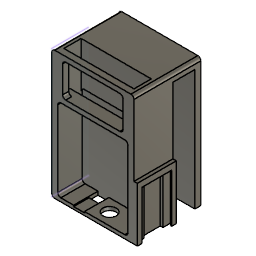
electronics_holder (Autodesk Fusion 360 design; units mm, degrees)
Autodesk Fusion 360 part; units mm, degrees
sketch "Sketch1" plane through (0, 0, 0) normal (0, 0, 1) x (1, 0, 0)
  line L0 (28.775, -7.5) -> (-28.775, -7.5)
  line L1 (-28.775, -7.5) -> (-28.775, 7.5)
  line L2 (-28.775, 7.5) -> (28.775, 7.5)
  line L3 (28.775, 7.5) -> (28.775, -7.5)
  line L4 (28.775, -7.5) -> (-28.775, 7.5) construction
  line L5 (-28.775, -7.5) -> (28.775, 7.5) construction
  line L6 (33.775, -17.5) -> (-33.775, -17.5)
  line L7 (-33.775, -17.5) -> (-33.775, 17.5)
  line L8 (-33.775, 17.5) -> (33.775, 17.5)
  line L9 (33.775, 17.5) -> (33.775, -17.5)
  line L10 (33.775, -17.5) -> (-33.775, 17.5) construction
  line L11 (-33.775, -17.5) -> (33.775, 17.5) construction
  line L12 (-28.775, -7.5) -> (-28.775, -17.5)
  line L13 (28.775, -7.5) -> (28.775, -17.5)
  line L14 (33.775, -7.5) -> (-33.775, -7.5)
  dimension "d1" = 57.55
  dimension "d2" = 15
  dimension "d3" = 10
  dimension "d4" = 5
  constraint horizontal L0
  constraint perpendicular L0 L1
  constraint parallel L0 L2
  constraint parallel L1 L3
  constraint coincident L4 origin
  constraint coincident L5 origin
  constraint horizontal L6
  constraint perpendicular L6 L7
  constraint parallel L6 L8
  constraint parallel L7 L9
  constraint coincident L10 origin
  constraint coincident L11 origin
  constraint coincident L6 L12.end
  constraint perpendicular L6 L12
  constraint coincident L6 L13.end
  constraint perpendicular L6 L13
  constraint coincident L9 L14.start
  constraint coincident L7 L14.end
  constraint perpendicular L7 L14
  measures "d1" distance of L1.end L2.end
  measures "d2" distance of L0.start L2.end
  measures "d3" distance of L2 L8
  measures "d4" distance of L3 L9
extrude "Extrude1" add sketch "Sketch1" against normal blind 5 contours L0 L1 L2 L3 L14 | L1 L2 L3 L7 L8 L9 L14 makes body 1
extrude "Extrude2" add sketch "Sketch1" along normal blind 65.5 contours L1 L2 L3 L7 L8 L9 L14 bodies 1
sketch "Sketch2" plane through (0, 0, 0) normal (0, 0, 1) x (-1, 0, 0)
  line L0 (-28.775, 7.5) -> (-28.775, -7.5)
  line L1 (-28.775, -7.5) -> (28.775, -7.5)
  line L2 (28.775, -7.5) -> (28.775, 7.5)
  line L3 (28.775, 2.5) -> (-28.775, 2.5) construction
  circle A0 centre (-3.775, 2.5) radius 5.25
  line L4 (28.775, 7.5) -> (-28.775, 7.5)
  dimension "d9" = 10.5
  dimension "d10" = 25
  dimension "d11" = 10
  constraint coincident L2 L3.start
  constraint coincident L0 L3.end
  constraint perpendicular L0 L3
  constraint coincident L3 A0.centre
  measures "d9" diameter of A0
  measures "d10" distance of L0 A0.centre
  measures "d11" distance of L1 A0.centre
extrude "Extrude3" cut sketch "Sketch2" against normal blind 10 contours A0 L4 | A0 L4 bodies 1
sketch "Sketch3" plane through (0, 0, 0) normal (0, 0, 1) x (-1, 0, 0)
  line L0 (-28.775, 7.5) -> (-28.775, -7.5)
  line L1 (-28.775, -7.5) -> (28.775, -7.5)
  line L2 (28.775, -7.5) -> (28.775, 7.5)
  line L3 (6.775, -7.5) -> (6.775, -0.1264)
  line L4 (6.775, -0.1264) -> (15.775, -0.1264)
  line L5 (15.775, -0.1264) -> (15.775, -7.5)
  line L6 (28.775, 7.5) -> (-2.1742, 7.5)
  line L7 (-5.3758, 7.5) -> (-28.775, 7.5)
  arc A0 (-5.3758, 7.5) -> (-2.1742, 7.5) centre (-3.775, 2.5) ccw
  dimension "d14" = 13
  dimension "d15" = 9
  constraint coincident L1 L3.start
  constraint perpendicular L1 L3
  constraint perpendicular L3 L4
  constraint coincident L1 L5.end
  constraint perpendicular L1 L5
  measures "d14" distance of L2 L5
  measures "d15" distance of L3.end L4.end
extrude "Extrude4" cut sketch "Sketch3" against normal blind 6 contours L1 L3 L4 L5 bodies 1
sketch "Sketch4" plane through (28.775, 0, 0) normal (-1, 0, 0) x (0, -1, 0)
  line L0 (-7.5, 0) -> (7.5, 0)
  line L1 (7.5, 65.5) -> (-7.5, 65.5)
  line L2 (-7.5, 65.5) -> (-7.5, 0)
  line L3 (-17.5, 65.5) -> (-12.5, 100.5)
  line L4 (-12.5, 100.5) -> (-1.5, 100.5)
  line L5 (-1.5, 100.5) -> (-1.5, 65.5)
  line L6 (-17.5, 65.5) -> (-1.5, 65.5)
  line L7 (7.5, 0) -> (7.5, 65.5)
  point P0 (-17.5, 65.5)
  dimension "d19" = 6
  dimension "d20" = 35
  constraint perpendicular L2 L4
  constraint coincident P0 L3.start
  constraint coincident L1 L5.end
  constraint perpendicular L1 L5
  measures "d19" distance of L1.end L5.end
  measures "d20" distance of L4.end L5.end
extrude "Extrude5" add sketch "Sketch4" along normal blind 57.55 separate body contours L1 L3 L4 L5 L6 makes body 2
extrude "Extrude6" add 1 faces at (9.5917, 14.1667, 65.5) along direction (0, 0, 1) blind 35 on bodies 1 bodies 1 2
sketch "Sketch6" plane through (0, -7.5, 0) normal (0, -1, 0) x (1, 0, 0)
  line L0 (28.775, 0) -> (-28.775, 0)
  line L1 (-28.775, 0) -> (-28.775, 100.5)
  line L2 (-28.775, 100.5) -> (-33.775, 100.5)
  line L3 (-33.775, 100.5) -> (-33.775, -5)
  line L4 (-33.775, -5) -> (33.775, -5)
  line L5 (33.775, -5) -> (33.775, 100.5)
  line L6 (33.775, 100.5) -> (28.775, 100.5)
  line L7 (28.775, 100.5) -> (28.775, 0)
  line L8 (28.775, 65.5) -> (28.775, 100.5)
  line L9 (28.775, 100.5) -> (-28.775, 100.5)
  line L10 (-28.775, 100.5) -> (-28.775, 65.5)
  line L11 (-28.775, 65.5) -> (28.775, 65.5)
  line L12 (-28.775, 100.5) -> (28.775, 65.5) construction
  line L13 (24.775, 69.5) -> (-24.775, 69.5)
  line L14 (-24.775, 69.5) -> (-24.775, 96.5)
  line L15 (-24.775, 96.5) -> (24.775, 96.5)
  line L16 (24.775, 96.5) -> (24.775, 69.5)
  line L17 (24.775, 69.5) -> (-24.775, 96.5) construction
  line L18 (-24.775, 69.5) -> (24.775, 96.5) construction
  line L19 (5.3758, -5) -> (33.775, -5)
  line L20 (33.775, -5) -> (33.775, 100.5)
  line L21 (33.775, 100.5) -> (28.775, 100.5)
  line L22 (28.775, 100.5) -> (28.775, 0)
  line L23 (28.775, 0) -> (5.3758, 0)
  line L24 (5.3758, 0) -> (5.3758, -5)
  point P0 (0, 83)
  dimension "d27" = 4
  dimension "d28" = 4
  constraint coincident L1.end L2.start
  constraint coincident L8.start L11.end
  constraint horizontal L13
  constraint perpendicular L13 L14
  constraint parallel L13 L15
  constraint parallel L14 L16
  constraint coincident L17 P0
  constraint coincident L18 P0
  constraint midpoint L12 P0
  measures "d27" distance of L9 L15
  measures "d28" distance of L7 L16
extrude "Extrude7" add sketch "Sketch6" along normal blind 5 contours L0 L4 L5 L6 L7 L8 L19 L20 L21 L22 L23 L24 | L0 L1 L2 L3 L4 L10 L24 | L1 L7 L8 L9 L10 L11 L22 bodies 1
sketch "Sketch15" plane through (0, -7.5, 0) normal (0, 1, 0) x (-1, 0, 0)
  line L0 (-28.775, 100.5) -> (-28.775, 65.5)
  line L1 (-28.775, 65.5) -> (28.775, 65.5)
  line L2 (28.775, 65.5) -> (28.775, 100.5)
  line L3 (28.775, 100.5) -> (-28.775, 100.5)
  line L4 (-24.775, 96.5) -> (24.775, 96.5)
  line L5 (24.775, 96.5) -> (24.775, 69.5)
  line L6 (24.775, 69.5) -> (-24.775, 69.5)
  line L7 (-24.775, 69.5) -> (-24.775, 96.5)
  line L8 (-24.775, 69.5) -> (-28.775, 69.5)
  line L9 (-28.775, 69.5) -> (28.775, 69.5)
  constraint coincident L6.end L7.start
  constraint coincident L0 L8.end
  constraint perpendicular L0 L8
  constraint coincident L2 L9.end
  constraint perpendicular L2 L9
extrude "Extrude17" add sketch "Sketch15" along normal blind 5 contours L0 L1 L2 L6 L8 L9 bodies 1
fillet "Fillet1" radius 2.5 10 edges at (-24.775, -10, 96.5) (-24.775, -10, 69.5) (24.775, -10, 69.5) (24.775, -10, 96.5) (-28.775, 4.5, 65.5) (-28.775, -10, 65.5) (-28.775, -2.5, 0) (28.775, -2.5, 0) (28.775, -10, 65.5) (28.775, 4.5, 65.5) on bodies 1
sketch "Sketch7" plane through (33.775, 0, 0) normal (1, 0, 0) x (0, 1, 0)
  line L0 (17.5, -5) -> (17.5, 100.5)
  line L1 (-12.5, 100.5) -> (-12.5, -5)
  line L2 (2.5, -4.4234) -> (2.5, 39.7315) construction
  line L3 (-11.625, 39.7315) -> (16.625, 39.7315)
  line L4 (-11.625, 39.7315) -> (-11.625, -5)
  line L5 (16.625, 39.7315) -> (16.618, -5)
  line L6 (-11.625, 39.7315) -> (-12.5, 39.7315)
  line L7 (16.625, 39.7315) -> (17.5, 39.7315)
  line L8 (-12.5, 37) -> (17.5, 37)
  line L9 (-12.5, -5) -> (17.5, -5)
  line L10 (17.5, 100.5) -> (-12.5, 100.5)
  point P0 (2.5, 37)
  dimension "d35" = 28.25
  dimension "d44" = 42
  constraint midpoint L2.end L3
  constraint perpendicular L2 L3
  constraint perpendicular L3 L4
  constraint coincident L1 L6.end
  constraint perpendicular L1 L6
  constraint coincident L0 L7.end
  constraint perpendicular L0 L7
  constraint midpoint L8 P0
  constraint coincident L2 P0
  constraint coincident L0 L8.end
  constraint perpendicular L0 L8
  constraint vertical L2
  constraint coincident L4.end L9
  constraint coincident L5.end L9
  measures "d35" distance of L3.start L3.end
  measures "d44" distance of L8 L9
extrude "Extrude9" add sketch "Sketch7" along normal blind 1.8 contours L0 L5 L8 L9 | L0 L5 L7 L8 | L3 L4 L5 L8 | L1 L4 L8 L9 | L1 L4 L6 L8 bodies 1
sketch "Sketch8" plane through (35.575, 0, 0) normal (1, 0, 0) x (0, 1, 0)
  line L0 (17.5, 39.7315) -> (-12.5, 39.7315)
  line L1 (-12.5, 39.7315) -> (-12.5, -5)
  line L2 (-11.625, -5) -> (-11.625, 37)
  line L3 (-11.625, 37) -> (16.6246, 37)
  line L4 (16.6246, 37) -> (16.618, -5)
  line L5 (17.5, -5) -> (17.5, 39.7315)
  line L6 (-9.6187, 35.0038) -> (14.6243, 35)
  line L7 (-12.5, -5) -> (-11.625, -5)
  line L8 (16.618, -5) -> (17.5, -5)
  line L9 (14.6243, 35) -> (14.618, -5)
  line L10 (-9.6187, 35.0038) -> (-9.625, -5.0074)
  line L11 (17.5, -5) -> (17.5, 39.7315)
  line L12 (17.5, 39.7315) -> (-12.5, 39.7315)
  line L13 (-12.5, 39.7315) -> (-12.5, -5)
  line L14 (-12.5, -5) -> (-11.625, -5)
  line L15 (-11.625, -5) -> (-11.625, 37)
  line L16 (-11.625, 37) -> (16.6246, 37)
  line L17 (16.6246, 37) -> (16.618, -5)
  line L18 (16.618, -5) -> (17.5, -5)
  line L19 (16.618, -5) -> (-11.625, -5)
  dimension "d45" = 2
  dimension "d46" = 2
  dimension "d47" = 2
  constraint perpendicular L4 L6
  constraint perpendicular L6 L9
  constraint perpendicular L6 L10
  constraint coincident L9.end L19
  measures "d45" horizontal distance of L2.start L10.end
  measures "d46" distance of L9.end L4.end
  measures "d47" vertical distance of L6.end L3.end
sketch "Sketch9" plane through (-33.775, 0, 0) normal (-1, 0, 0) x (0, -1, 0)
  line L0 (12.5, -5) -> (12.5, 100.5)
  line L1 (-17.5, 100.5) -> (-17.5, -5)
  line L2 (-17.5, -5) -> (12.5, -5)
  line L3 (12.5, 100.5) -> (-17.5, 100.5)
sketch "Sketch10" plane through (-33.775, 0, 0) normal (-1, 0, 0) x (0, -1, 0)
  line L0 (-17.5, 100.5) -> (-17.5, -5)
  line L1 (-17.5, -5) -> (-37.5, -5)
  line L2 (-37.5, -5) -> (-37.5, 1.25)
  line L3 (-37.5, 1.25) -> (-19.5, 1.25)
  line L4 (-19.5, 1.25) -> (-19.5, 94.25)
  line L5 (-19.5, 94.25) -> (-37.5, 94.25)
  line L6 (-37.5, 94.25) -> (-37.5, 100.5)
  line L7 (-37.5, 100.5) -> (-17.5, 100.5)
  dimension "d48" = 2
  dimension "d49" = 93
  dimension "d50" = 18
  constraint coincident L0.end L1.start
  constraint perpendicular L0 L1
  constraint perpendicular L1 L2
  constraint perpendicular L2 L3
  constraint perpendicular L3 L4
  constraint perpendicular L4 L5
  constraint perpendicular L5 L6
  constraint coincident L0.start L7.end
  constraint perpendicular L0 L7
  constraint equal L2 L6
  constraint equal L3 L5
  measures "d48" distance of L0 L4
  measures "d49" distance of L3.end L4.end
  measures "d50" distance of L2.end L3.end
extrude "Extrude11" add sketch "Sketch10" against normal blind 67.55 bodies 1
sketch "Sketch11" plane through (-33.775, 0, 0) normal (-1, 0, 0) x (0, -1, 0)
  line L0 (-37.5, -5) -> (12.5, -5)
  line L1 (12.5, -5) -> (12.5, 100.5)
  line L2 (12.5, 100.5) -> (-37.5, 100.5)
  line L3 (-37.5, 100.5) -> (-37.5, 94.25)
  line L4 (-37.5, 94.25) -> (-19.5, 94.25)
  line L5 (-19.5, 94.25) -> (-19.5, 1.25)
  line L6 (-19.5, 1.25) -> (-37.5, 1.25)
  line L7 (-37.5, 1.25) -> (-37.5, -5)
  line L8 (-37.5, 1.25) -> (-37.5, 94.25)
  constraint coincident L6.end L7.start
  constraint coincident L3.end L4.start
extrude "Extrude12" add sketch "Sketch11" against normal blind 5 contours L4 L5 L6 L8 bodies 1
sketch "Sketch12" plane through (33.775, 0, 0) normal (1, 0, 0) x (0, 1, 0)
  line L0 (-12.5, 39.7315) -> (17.5, 39.7315)
  line L1 (17.5, 39.7315) -> (17.5, -5)
  line L2 (17.5, -5) -> (37.5, -5)
  line L3 (37.5, -5) -> (37.5, 1.25)
  line L4 (37.5, 1.25) -> (19.5, 1.25)
  line L5 (19.5, 1.25) -> (19.5, 94.25)
  line L6 (19.5, 94.25) -> (37.5, 94.25)
  line L7 (37.5, 94.25) -> (37.5, 100.5)
  line L8 (37.5, 100.5) -> (-12.5, 100.5)
  line L9 (-12.5, 100.5) -> (-12.5, 39.7315)
  line L10 (19.5, 1.25) -> (17.5, 1.25)
  constraint coincident L4.end L5.start
  constraint coincident L1 L10.end
  constraint perpendicular L1 L10
extrude "Extrude13" cut sketch "Sketch12" against normal blind 19 contours L1 L2 L3 L4 L10 bodies 1
extrude "Extrude14" add 1 faces at (27.4417, 18.8333, 1.25) along direction (0, 0, -1) blind 6.25 on bodies 1 bodies 1
sketch "Sketch13" plane through (0, 37.5, 0) normal (0, 1, 0) x (-1, 0, 0)
  line L0 (-14.775, 1.25) -> (-14.775, -5)
  line L1 (-14.775, -5) -> (33.775, -5)
  line L2 (33.775, -5) -> (33.775, 100.5)
  line L3 (33.775, 100.5) -> (-33.775, 100.5)
  line L4 (-33.775, 100.5) -> (-33.775, 94.25)
  line L5 (-33.775, 94.25) -> (28.775, 94.25)
  line L6 (28.775, 94.25) -> (28.775, 1.25)
  line L7 (28.775, 1.25) -> (-14.775, 1.25)
  line L8 (-33.775, 94.25) -> (-33.775, -5)
  line L9 (-33.775, -5) -> (-14.775, -5)
  constraint coincident L4.end L5.start
  constraint perpendicular L5 L8
  constraint coincident L0.end L1.start
  constraint perpendicular L0 L9
extrude "Extrude15" add sketch "Sketch13" along normal blind 5 bodies 1
sketch "Sketch14" plane through (0, 0, -5) normal (0, 0, -1) x (1, 0, 0)
  line L0 (33.775, -17.5) -> (35.575, -17.5)
  line L1 (35.575, -16.618) -> (33.775, -16.618)
  line L2 (33.775, -16.618) -> (33.775, 11.625)
  line L3 (33.775, 11.625) -> (35.575, 11.625)
  line L4 (35.575, 12.5) -> (-33.775, 12.5)
  line L5 (-33.775, 12.5) -> (-33.775, -42.5)
  line L6 (-33.775, -42.5) -> (33.775, -42.5)
  line L7 (33.775, -37.5) -> (14.775, -37.5)
  line L8 (14.775, -37.5) -> (14.775, -19.5)
  line L9 (14.775, -19.5) -> (33.775, -19.5)
  arc A0 (2.1742, 7.5) -> (5.3758, 7.5) centre (3.775, 2.5) ccw
  line L10 (2.1742, 7.5) -> (5.3758, 7.5)
  line L11 (-15.775, -7.5) -> (-15.775, -0.1264)
  line L12 (-15.775, -0.1264) -> (-6.775, -0.1264)
  line L13 (-6.775, -0.1264) -> (-6.775, -7.5)
  line L14 (-6.775, -7.5) -> (-15.775, -7.5)
  circle A1 centre (3.775, 2.5) radius 5.5
  line L15 (35.575, -17.5) -> (35.575, -16.618)
  line L16 (35.575, 11.625) -> (35.575, 12.5)
  line L17 (33.775, -42.5) -> (33.775, -37.5)
  line L18 (33.775, -19.5) -> (33.775, -17.5)
  dimension "d61" = 11
  constraint concentric A0 A1
  measures "d61" diameter of A1
extrude "Extrude16" cut sketch "Sketch14" against normal blind 5 contours A1 bodies 1
extrude "Extrude18" cut 1 faces at (8.7583, 1.5, 88.8333) along direction (0, 1, 0) blind 5.2 on bodies 1 bodies 1
delete_face "DeleteFace1" 1 faces at (26.8644, -5.8333, 0.0705) on bodies 1
delete_face "DeleteFace2" 1 faces at (-28.7637, -5.8333, 2.2624) on bodies 1
extrude "Extrude19" cut 1 faces at (22.275, -2.5, 0) along direction (0, 0, -1) blind 2 on bodies 1 bodies 1
extrude "Extrude20" add 1 faces at (34.975, 17.5, 24.821) along direction (0, 1, 0) blind 2 and the other way blind 30 on bodies 1 bodies 1
sketch "Sketch16" plane through (35.575, 0, 0) normal (1, 0, 0) x (0, 1, 0)
  line L0 (19.5, 39.7315) -> (-12.5, 39.7315)
  line L1 (-12.5, 39.7315) -> (-12.5, -5)
  line L2 (-12.5, -5) -> (19.5, -5)
  line L3 (19.5, -5) -> (19.5, 39.7315)
  line L4 (3.5, -5) -> (3.5, 37) construction
  line L5 (-10.65, 37) -> (17.65, 37)
  line L6 (-10.65, 37) -> (-10.65, -5)
  line L7 (17.65, 37) -> (17.65, -5)
  dimension "d76" = 42
  dimension "d77" = 28.3
  constraint midpoint L2 L4.start
  constraint perpendicular L2 L4
  constraint midpoint L4.end L5
  constraint perpendicular L3 L5
  constraint coincident L2 L6.end
  constraint perpendicular L2 L6
  constraint coincident L2 L7.end
  constraint perpendicular L2 L7
  measures "d76" distance of L4.start L4.end
  measures "d77" distance of L5.start L5.end
extrude "Extrude21" cut sketch "Sketch16" against normal blind 1.75 contours L2 L5 L6 L7 bodies 1
sketch "Sketch17" plane through (33.825, 0, 0) normal (1, 0, 0) x (0, 1, 0)
  line L0 (-10.65, 37) -> (-10.65, -5)
  line L1 (-10.65, -5) -> (17.65, -5)
  line L2 (17.65, -5) -> (17.65, 37)
  line L3 (17.65, 37) -> (-10.65, 37)
  line L4 (3.5, -5) -> (3.5, 37)
  line L5 (-4.25, 37) -> (11.25, 37)
  line L6 (-4.25, 37) -> (-4.25, -5)
  line L7 (11.25, 37) -> (11.25, -5)
  dimension "d80" = 15.5
  constraint midpoint L1 L4.start
  constraint perpendicular L1 L4
  constraint midpoint L4.end L5
  constraint perpendicular L4 L5
  constraint coincident L1 L6.end
  constraint perpendicular L1 L6
  constraint coincident L1 L7.end
  constraint perpendicular L1 L7
  constraint collinear L3 L5
  measures "d80" distance of L5.start L5.end
extrude "Extrude22" cut sketch "Sketch17" against normal blind 2 contours L1 L3 L4 L5 L6 | L1 L3 L4 L5 L7 bodies 1
sketch "Sketch18" plane through (35.575, 0, 0) normal (1, 0, 0) x (0, 1, 0)
  line L0 (-10.65, -5) -> (-10.65, 37)
  line L1 (-10.65, 37) -> (17.65, 37)
  line L2 (17.65, 37) -> (17.65, -5)
  line L3 (17.65, -5) -> (19.5, -5)
  line L4 (19.5, -5) -> (19.5, 39.7315)
  line L5 (19.5, 39.7315) -> (-12.5, 39.7315)
  line L6 (-12.5, 39.7315) -> (-12.5, -5)
  line L7 (-12.5, -5) -> (-10.65, -5)
  line L8 (-10.65, -5) -> (-8.65, -5)
  line L9 (-8.65, -5) -> (-8.65, 35)
  line L10 (-8.65, 35) -> (15.65, 35)
  line L11 (15.65, 35) -> (15.65, -5)
  line L12 (15.65, -5) -> (17.65, -5)
  dimension "d83" = 2
  dimension "d84" = 2
  dimension "d85" = 2
  constraint coincident L0.start L7.end
  constraint perpendicular L0 L8
  constraint perpendicular L8 L9
  constraint perpendicular L0 L10
  constraint coincident L2.end L3.start
  constraint vertical L11
  measures "d83" distance of L0 L9
  measures "d84" distance of L1 L10
  measures "d85" distance of L2 L11
extrude "Extrude23" add sketch "Sketch18" along normal blind 1 bodies 1
fillet "Fillet4" radius 2.5 2 edges at (28.775, -2.5, -2) (-28.775, -2.5, -2) on bodies 1
fillet "Fillet5" radius 2.5 3 edges at (-33.775, 15, 100.5) (-33.775, 15, -5) (33.775, 15, 100.5) on bodies 1
sketch "Sketch19" plane through (0, -12.5, 0) normal (0, -1, 0) x (1, 0, 0)
  arc A0 (33.775, 98) -> (31.275, 100.5) centre (31.275, 98) ccw
  line L0 (31.275, 100.5) -> (-31.275, 100.5)
  arc A1 (-31.275, 100.5) -> (-33.775, 98) centre (-31.275, 98) ccw
  line L1 (-33.775, 98) -> (-33.775, -2.5)
  arc A2 (-33.775, -2.5) -> (-31.275, -5) centre (-31.275, -2.5) ccw
  line L2 (-31.275, -5) -> (36.575, -5)
  line L3 (36.575, -5) -> (36.575, 39.7315)
  line L4 (36.575, 39.7315) -> (33.775, 39.7315)
  line L5 (33.775, 39.7315) -> (33.775, 98)
  line L6 (-28.775, 0.5) -> (-28.775, 63)
  arc A3 (-26.275, 65.5) -> (-28.775, 63) centre (-26.275, 63) ccw
  line L7 (-26.275, 65.5) -> (26.275, 65.5)
  arc A4 (28.775, 63) -> (26.275, 65.5) centre (26.275, 63) ccw
  line L8 (28.775, 63) -> (28.775, 0.5)
  arc A5 (26.275, -2) -> (28.775, 0.5) centre (26.275, 0.5) ccw
  line L9 (26.275, -2) -> (-26.275, -2)
  arc A6 (-28.775, 0.5) -> (-26.275, -2) centre (-26.275, 0.5) ccw
  line L10 (-22.275, 96.5) -> (22.275, 96.5)
  arc A7 (24.775, 94) -> (22.275, 96.5) centre (22.275, 94) ccw
  line L11 (24.775, 94) -> (24.775, 72)
  arc A8 (22.275, 69.5) -> (24.775, 72) centre (22.275, 72) ccw
  line L12 (22.275, 69.5) -> (-22.275, 69.5)
  arc A9 (-24.775, 72) -> (-22.275, 69.5) centre (-22.275, 72) ccw
  line L13 (-24.775, 72) -> (-24.775, 94)
  arc A10 (-22.275, 96.5) -> (-24.775, 94) centre (-22.275, 94) ccw
  line L14 (-15.775, -5) -> (-6.775, -5)
  line L15 (-15.775, -2) -> (-6.8347, -2)
  line L16 (-15.775, -2) -> (-15.775, -3)
  line L17 (-15.775, -3) -> (-6.8347, -3)
  line L18 (-6.8347, -3) -> (-6.8347, -2)
  constraint coincident L9 L15.start
  constraint coincident L9 L15.end
  constraint perpendicular L9 L16
  constraint perpendicular L16 L17
  constraint perpendicular L9 L18
extrude "Extrude24" cut sketch "Sketch19" against normal blind 20 contours L9 L15 L16 L17 L18 bodies 1
extrude "Extrude25" cut 1 faces at (31.825, 6.0833, 9) along direction (-1, 0, 0) blind 0.2 on bodies 1 bodies 1
